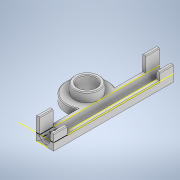
# Autodesk Inventor part: ipad holder
Saved by Autodesk Inventor 2020 (Build 240168000, 168)
## iProperties
Created: 2020-05-17
Part Number: ipad holder
Material: Generic
Document SubType Name: Modeling
Designer: maxde
Density: 1 g/cm^3
Appearance: Default
Author: maxde
Autodesk Inventor part; units mm, degrees
ref_plane "YZ Plane" through (0, 0, 0) normal (1, 0, 0) x (0, 1, 0)
ref_plane "XZ Plane" through (0, 0, 0) normal (0, 1, 0) x (-1, 0, 0)
ref_plane "XY Plane" through (0, 0, 0) normal (0, 0, 1) x (1, 0, 0)
sketch "Sketch1" plane through (0, 0, 0) normal (0, 1, 0) x (-1, 0, 0)
  circle A0 centre (0, 0) radius 13.8
  circle A1 centre (0, 0) radius 5
  circle A2 centre (0, 0) radius 6
  dimension "d0" = 27.6
  dimension "d1" = 10
  dimension "d2" = 12
  constraints: 3 centre point, 3 coincident
  measures "d0" diameter of A0
  measures "d1" diameter of A1
  measures "d2" diameter of A2
extrude "Extrusion1" add sketch "Sketch1" along normal blind 5 contours A0
sketch "Sketch2" plane through (0, 0, 0) normal (0, -1, 0) x (1, 0, 0)
  circle A0 centre (0, 0) radius 6 projected
  line L0 (6, 0) -> (13.8, 0)
  circle A1 centre (0, 0) radius 13.8 projected
  line L1 (13.8, -40) -> (6, -40)
  line L2 (6, -40) -> (6, 40)
  line L3 (6, 40) -> (13.8, 40)
  line L4 (13.8, 40) -> (13.8, -40)
  line L5 (13.8, -40) -> (6, 40) construction
  line L6 (6, -40) -> (13.8, 40) construction
  line L7 (17.7, 40) -> (9.9, 40)
  line L8 (9.9, 40) -> (9.9, -40)
  line L9 (9.9, -40) -> (17.7, -40)
  line L10 (17.7, -40) -> (17.7, 40)
  line L11 (17.7, 40) -> (9.9, -40) construction
  line L12 (9.9, 40) -> (17.7, -40) construction
  point P0 (9.9, 0)
  point P1 (6, -12.4274)
  point P2 (6, 12.4274)
  dimension "d5" = 80
  constraints: 26 end point, 6 midpoint, 4 parallel, 3 horizontal, 2 perpendicular, 1 horizontal alignment, 3 other
  measures "d5" distance of L1.end L2.end
extrude "Extrusion2" add sketch "Sketch2" against normal blind 5 contours A1 L8 L1 L2 | L2 L3 L8 A1 | L4 L1 L8 A1 | A1 L8 L3 L4 | L4 L7 L10 L9
sketch "Sketch3" plane through (6, 0, 40) normal (0, 0, 1) x (1, 0, 0)
  line L0 (-12, 5) -> (0, 5) projected
  line L1 (7.8, 0) -> (0, 0) projected
  line L2 (0, 5) -> (7.8, 0) construction
  line L3 (0, 5) -> (7.8, 5) construction
  line L4 (0, 0) -> (7.8, 5) construction
  point P0 (-6, 0)
  constraints: 4 end point
sketch "Sketch4" plane through (6, 0, 40) normal (0, 0, 1) x (1, 0, 0)
  line L0 (0, 0) -> (0, 5) projected
  line L1 (0, 2.5) -> (11.7, 2.5)
  line L2 (11.7, 0) -> (11.7, 5) projected
  line L3 (5.85, 2.5) -> (5.85, 5)
  line L4 (0, 5) -> (11.7, 5) projected
  circle A0 centre (5.85, 5) radius 3.5
  point P0 (-6, 0)
  point P1 (2.35, 5)
  point P2 (9.35, 5)
  dimension "d8" = 7
  constraints: 4 end point, 4 midpoint, 1 centre point, 1 coincident
  measures "d8" diameter of A0
extrude "Extrusion3" cut sketch "Sketch4" against normal through all contours A0 L4 L3 L1 | L1 A0 | L3 L4 A0 L1
sketch "Sketch5" plane through (0, 5, 0) normal (0, 1, 0) x (1, 0, 0)
  line L0 (17.7, -40) -> (6, -40) projected
  line L1 (8.35, -40) -> (8.35, 40) projected
  line L2 (6, -40) -> (8.35, -40)
  line L3 (8.35, -40) -> (8.35, -31)
  line L4 (8.35, -31) -> (6, -31)
  line L5 (6, -31) -> (6, -40)
  line L6 (15.35, 40) -> (15.35, -40) projected
  line L7 (17.7, -40) -> (17.7, 40) projected
  line L8 (15.35, -40) -> (17.7, -40)
  line L9 (17.7, -40) -> (17.7, -31)
  line L10 (17.7, -31) -> (15.35, -31)
  line L11 (15.35, -31) -> (15.35, -40)
  point P0 (0, 0)
  dimension "d11" = 9
  constraints: 16 end point, 4 parallel, 2 horizontal, 2 perpendicular, 2 point on line
  measures "d11" distance of L3.end L2.end
extrude "Extrusion4" add sketch "Sketch5" along normal blind 10 contours L0 L5 L4 L1
extrude "Extrusion5" add sketch "Sketch5" along normal blind 5 contours L0 L6 L10 L7
mirror "Mirror1" about plane through (0, 0, 0) normal (0, 0, 1) of "Extrusion4", "Extrusion5"
sketch "Sketch6" plane through (0, 5, 0) normal (0, 1, 0) x (1, 0, 0)
  circle A0 centre (0, 0) radius 8.35
  circle A1 centre (0, 0) radius 6
  constraints: 2 centre point, 2 coincident
extrude "Extrusion6" add sketch "Sketch6" along normal blind 6
chamfer "Chamfer1" distance 0.5 angle 45 14 edges at (-8.35, 11, 0) (-6, 11, 0) (-13.8, 5, 0) (6, 5, -21.7137) (6, 5, 21.7137) (8.35, 15, 35.5) (6, 15, 35.5) (8.35, 15, -35.5) (6, 15, -35.5) (17.7, 10, -35.5) (15.35, 10, -35.5) (17.7, 10, 35.5) (15.35, 10, 35.5) (17.7, 5, 0)
body "Solid1"
